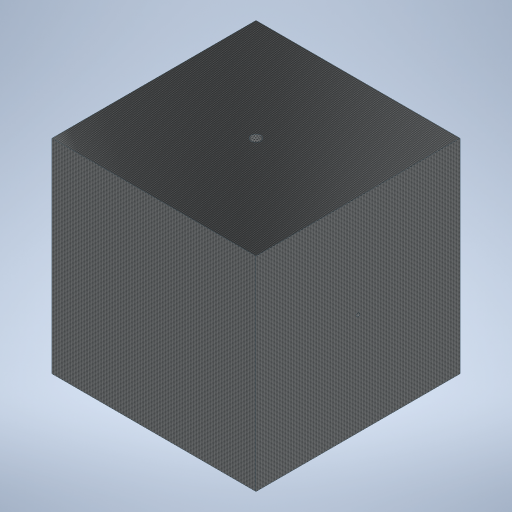
# Autodesk Inventor part: temporary
Saved by Autodesk Inventor 2024 (Build 280153000, 153)
## iProperties
Created: 2023-04-11
Part Number: temporary
Material: PC/ABS Plastic
Document SubType Name: Modeling
Designer: ASUS
Density: 0.357273 g/cm^3
Appearance: Expanded Metal 01
Author: ASUS
Autodesk Inventor part; units mm, degrees
ref_plane "YZ Plane" through (0, 0, 0) normal (1, 0, 0) x (0, 1, 0)
ref_plane "XZ Plane" through (0, 0, 0) normal (0, 1, 0) x (-1, 0, 0)
ref_plane "XY Plane" through (0, 0, 0) normal (0, 0, 1) x (1, 0, 0)
sketch "Sketch1" plane through (0, 0, 0) normal (0, 1, 0) x (-1, 0, 0)
  line L0 (0, 0) -> (300, 0)
  line L1 (300, 0) -> (300, -300)
  line L2 (300, -300) -> (0, -300)
  line L3 (0, -300) -> (0, 0)
  dimension "d0" = 300
  dimension "d1" = 300
  constraints: 8 end point, 2 parallel, 1 horizontal, 1 perpendicular
  measures "d0" distance of L1.end L2.end
  measures "d1" distance between parallel lines of L2 L0
extrude "Extrusion1" add sketch "Sketch1" along normal blind 300
sketch "Sketch3" plane through (0, 0, 0) normal (0, -1, 0) x (1, 0, 0)
  line L0 (-10, -270) -> (-280, -270)
  line L1 (-280, -270) -> (-280, -30)
  line L2 (-280, -30) -> (-10, -30)
  line L3 (-10, -30) -> (-10, -270)
  line L4 (0, 0) -> (0, -300) projected
  line L5 (-300, -300) -> (-300, 0) projected
  line L6 (0, -300) -> (-300, -300) projected
  line L7 (-300, 0) -> (0, 0) projected
  dimension "d10" = 10
  dimension "d11" = 20
  dimension "d12" = 30
  dimension "d13" = 30
  constraints: 8 end point, 2 parallel, 1 horizontal, 1 perpendicular
  measures "d10" distance between parallel lines of L4 L3
  measures "d11" distance between parallel lines of L5 L1
  measures "d12" distance between parallel lines of L6 L0
  measures "d13" distance between parallel lines of L7 L2
extrude "Extrusion3" cut sketch "Sketch3" against normal blind 10 contours L0 L1 L2 L3
sketch "Sketch5" plane through (-300, 0, -300) normal (-1, 0, 0) x (0, 0, 1)
  line L0 (10, 10) -> (290, 10)
  line L1 (290, 10) -> (290, 290)
  line L2 (290, 290) -> (10, 290)
  line L3 (10, 290) -> (10, 10)
  line L4 (0, 300) -> (300, 300) projected
  line L5 (0, 0) -> (300, 0) projected
  line L6 (0, 0) -> (0, 300) projected
  line L7 (300, 0) -> (300, 300) projected
  dimension "d22" = 10
  dimension "d23" = 10
  dimension "d24" = 10
  dimension "d25" = 10
  constraints: 8 end point, 2 parallel, 1 horizontal, 1 perpendicular
  measures "d22" distance between parallel lines of L2 L4
  measures "d23" distance between parallel lines of L5 L0
  measures "d24" distance between parallel lines of L6 L3
  measures "d25" distance between parallel lines of L7 L1
extrude "Extrusion5" cut sketch "Sketch5" against normal blind 290 contours L3 L2 L1 L0
sketch "Sketch7" plane through (0, 0, 0) normal (1, 0, 0) x (0, 0, -1)
  circle A0 centre (150, 150) radius 2.5
  line L0 (0, 300) -> (300, 300) projected
  line L1 (300, 0) -> (300, 300) projected
  point P0 (0, 0)
  dimension "d37" = 5
  dimension "d38" = 150
  dimension "d39" = 150
  constraints: 1 centre point
  measures "d37" diameter of A0
  measures "d38" distance from line of A0.centre L0
  measures "d39" distance from line of L1 A0.centre
extrude "Extrusion7" cut sketch "Sketch7" against normal blind 10
sketch "Sketch8" plane through (0, 300, 0) normal (0, 1, 0) x (1, 0, 0)
  circle A0 centre (-150, 150) radius 7.5
  line L0 (0, 0) -> (0, 300) projected
  line L1 (0, 300) -> (-300, 300) projected
  dimension "d42" = 15
  dimension "d43" = 150
  dimension "d44" = 150
  constraints: 1 centre point
  measures "d42" diameter of A0
  measures "d43" distance from line of A0.centre L0
  measures "d44" distance from line of L1 A0.centre
extrude "Extrusion8" cut sketch "Sketch8" against normal through all
body "Solid1"
